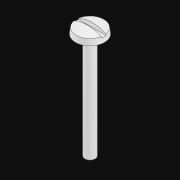
# Autodesk Inventor part: Screw 8-32 Nylon 1.250
Saved by Autodesk Inventor 2021.2 (Build 252289000, 289)
## iProperties
Created: 2020-07-03
Part Number: Screw 8-32 Nylon 1.250
Material: VEX Nylon
Document SubType Name: Modeling
Designer: yuany
Density: 1.12 g/cm^3
Appearance: Nylon 6
Author: yuany
Autodesk Inventor part; units mm, degrees
ref_plane "YZ Plane" through (0, 0, 0) normal (1, 0, 0) x (0, 1, 0)
ref_plane "XZ Plane" through (0, 0, 0) normal (0, 1, 0) x (-1, 0, 0)
ref_plane "XY Plane" through (0, 0, 0) normal (0, 0, 1) x (1, 0, 0)
sketch "Sketch1" plane through (0, 0, 0) normal (0, 1, 0) x (-1, 0, 0)
  circle A0 centre (0, 0) radius 1.5621
  dimension "d4" = 3.1242
  constraints: 1 centre point, 1 coincident
  measures "d4" diameter of A0
extrude "Body" add sketch "Sketch1" along normal blind 31.75
sketch "Sketch2" plane through (0, 0, 0) normal (1, 0, 0) x (0, 1, 0)
  line L0 (31.75, -1.5621) -> (31.75, 1.5621) projected
  line L1 (31.75, 0) -> (31.75, -4.3688)
  line L2 (33.4772, 0) -> (31.75, 0)
  line L3 (33.4772, 0) -> (33.4772, -4.1656)
  arc A0 (33.4772, -4.1656) -> (34.4169, 0) centre (24.7141, 0) ccw
  line L4 (31.75, -4.3688) -> (33.4772, -4.1656)
  line L5 (33.4772, 0) -> (34.4169, 0)
  point P0 (0, 0)
  dimension "d5" = 4.3688
  dimension "d13" = 1.7272
  dimension "d57" = 4.1656
  dimension "d58" = 9.7028
  dimension "d59" = 0
  constraints: 10 end point, 2 horizontal, 2 point on circle, 2 point on line, 1 centre point, 1 midpoint, 1 vertical
  measures "d5" distance of L1.start L1.end
  measures "d13" distance of L2.start L1.start
  measures "d57" distance of L2.start L3.end
  measures "d58" radius of A0
  measures "d59" distance from line of L2 A0.centre
revolve "Head" add sketch "Sketch2" angle 360 about axis through (0, 33.4772, 0) along (0, -1, 0)
sketch "Sketch6" plane through (0, 0, 0) normal (0, 0, 1) x (1, 0, 0)
  line L0 (0, 0) -> (-1.4859, 0)
  line L1 (1.5621, 0) -> (-1.5621, 0) projected
  line L2 (-1.4859, 0) -> (-2.4948, 1.0089)
  line L3 (-2.4948, 1.0089) -> (-2.9651, -1.2188)
  line L4 (-2.9651, -1.2188) -> (-1.4859, -1.2188)
  line L5 (-1.5621, 0) -> (-1.5621, 31.75) projected
  line L6 (-1.4859, -1.2188) -> (-1.4859, 0)
  line L7 (0, -3.9171) -> (0, 14.9707) projected
  point P0 (-1.5621, 0.0762)
  dimension "d49" = 1.4859
  dimension "d50" = 135
  constraints: 10 end point, 1 perpendicular, 1 point on line, 1 vertical
  measures "d49" distance from line of L0.start L6
  measures "d50" angle of L2 L6
revolve "Tapered End" cut sketch "Sketch6" angle 360 about axis through (0, -10, 0) along (0, 1, 0)
sketch "Sketch7" plane through (0, 0, 0) normal (1, 0, 0) x (0, 1, 0)
  line L0 (31.75, 4.3688) -> (31.75, -4.3688) projected
  line L1 (33.0962, 0.6985) -> (33.0962, -0.6985)
  line L2 (33.0962, 0.6985) -> (35.1028, 0.6985)
  line L3 (35.1028, 0.6985) -> (35.1028, -0.6985)
  line L4 (35.1028, -0.6985) -> (33.0962, -0.6985)
  point P0 (0, 0)
  dimension "d61" = 1.397
  dimension "d62" = 0.6985
  dimension "d65" = 33.0962
  dimension "d66" = 2.0066
  constraints: 8 end point, 1 horizontal, 1 parallel, 1 perpendicular, 1 vertical
  measures "d61" distance of L2.end L3.end
  measures "d62" distance from line of L2 point (0, 0)
  measures "d65" distance from line of point (0, 0) L1
  measures "d66" distance of L1.start L2.end
extrude "Flathead" cut sketch "Sketch7" against normal mid plane 12.7
body "Solid1"
